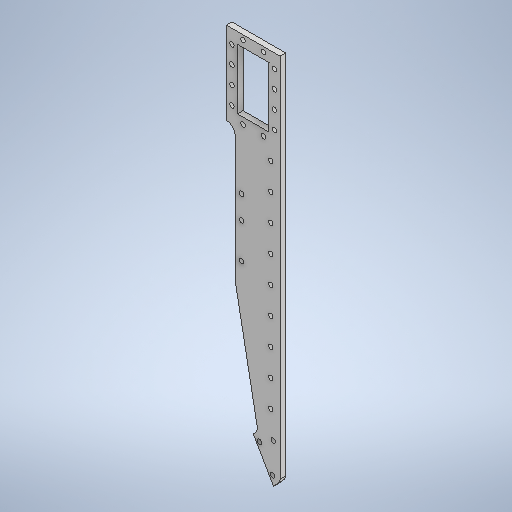
# Autodesk Inventor part: 1012
Saved by Autodesk Inventor 2025.1 (Build 291241000, 241)
## iProperties
Created: 2024-06-10
Part Number: 1012
Material: Generisch
Document SubType Name: Modeling
Designer: ffogue
Density: 1 g/cm^3
Appearance: Vorgabe
Author: ffogue
Autodesk Inventor part; units mm, degrees
ref_plane "XZ Plane" through (0, 0, 0) normal (0, 1, 0) x (-1, 0, 0)
sketch "Skizze1" plane through (0, 0, 0) normal (0, 1, 0) x (-1, 0, 0)
  line L0 (0, 0) -> (58, 0)
  line L1 (58, 0) -> (58, -89)
  arc A0 (58, -89) -> (48.5, -98.5) centre (58, -98.5) ccw
  line L2 (48.5, -98.5) -> (48.5, -218.5)
  line L3 (48.5, -218.5) -> (48.5, -234.2814)
  line L4 (0, 0) -> (0, -395.7321)
  line L5 (48.5, -218.5) -> (48.5, -250.0629) construction
  arc A1 (0, -395.7321) -> (1.4803, -399.6783) centre (6, -395.7321) ccw
  line L6 (1.4803, -399.6783) -> (7, -406)
  line L7 (7, -406) -> (29, -367.8949)
  line L8 (29, -367.8949) -> (29, -367.8949)
  arc A2 (24.7603, -358.6329) -> (29, -367.8949) centre (33.3956, -360.2814) ccw
  line L9 (24.7603, -358.6329) -> (48.5, -234.2814)
  line L10 (7, -406) -> (55.5885, -321.8422) construction
  dimension "d1" = 58
  dimension "d2" = 9.5
  dimension "d3" = 89
  dimension "d4" = 120
  dimension "d7" = 406
  dimension "d8" = 44
  dimension "d9" = 30
  dimension "d10" = 6
  dimension "d11" = 126
  dimension "d12" = 29
  dimension "d13" = 6
  constraints: 22 end point, 6 point on circle, 5 tangent, 3 centre point, 2 point on line, 2 vertical, 1 collinear, 1 horizontal, 1 midpoint, 1 parallel, 1 perpendicular
  measures "d1" distance of L0.start L0.end
  measures "d2" radius of A0
  measures "d3" distance of L0.end L1.end
  measures "d4" distance of L2.start L2.end
  measures "d7" vertical distance of L0.start L6.end
  measures "d8" distance of L6.end L7.end
  measures "d9" angle of L10 L5
  measures "d10" distance from line of A1.centre L10
  measures "d11" vertical distance of L3.end A2.centre
  measures "d12" distance from line of L4 L7.end
  measures "d13" distance from line of L4 A1.centre
extrude "Extrusion1" add sketch "Skizze1" along normal blind 6
sketch "Skizze2" plane through (0, 6, 0) normal (0, 1, 0) x (1, 0, 0)
  line L0 (-46, 12) -> (-12, 12)
  line L1 (-12, 12) -> (-12, 77)
  line L2 (-12, 77) -> (-46, 77)
  line L3 (-46, 77) -> (-46, 12)
  line L4 (-58, 0) -> (0, 0) projected
  point P0 (-29, 12)
  point P1 (-29, 0)
  dimension "d16" = 34
  dimension "d17" = 65
  dimension "d18" = 12
  constraints: 8 end point, 2 midpoint, 2 parallel, 1 horizontal, 1 perpendicular, 1 vertical alignment
  measures "d16" distance between parallel lines of L1 L3
  measures "d17" distance of L2.end L0.start
  measures "d18" distance between parallel lines of L4 L0
extrude "Extrusion2" cut sketch "Skizze2" against normal up to surface (6 mm away)
sketch "Skizze3" plane through (0, 6, 0) normal (0, 1, 0) x (1, 0, 0)
  line L0 (-58, 0) -> (0, 0) projected
  point P0 (-40, 5)
  point P1 (-18, 5)
  point P2 (-29, 0)
  point P3 (-29, 0)
  dimension "d21" = 11
  dimension "d22" = 11
  dimension "d23" = 5
  constraints: 2 midpoint, 1 horizontal alignment
  measures "d21" horizontal distance of point (-29, 0) point (-40, 5)
  measures "d22" horizontal distance of point (-29, 0) point (-18, 5)
  measures "d23" distance from line of L0 point (-18, 5)
hole "Bohrung1" at (-40, 6, -5) at (-18, 6, -5) direction (0, -1, 0) diameter 5 end through all
sketch "Skizze4" plane through (0, 6, 0) normal (0, 1, 0) x (1, 0, 0)
  circle A0 centre (-40, 5) radius 2.5 projected
  line L0 (-58, 89) -> (-58, 0) projected
  point P0 (0, 0)
  point P1 (-52, 15)
  point P2 (-52, 34)
  point P3 (-52, 53)
  point P4 (-52, 72)
  dimension "d31" = 10
  dimension "d32" = 19
  dimension "d33" = 19
  dimension "d34" = 19
  dimension "d35" = 6
  constraints: 3 vertical alignment
  measures "d31" vertical distance of point (-52, 15) A0.centre
  measures "d32" distance of point (-52, 34) point (-52, 15)
  measures "d33" distance of point (-52, 53) point (-52, 34)
  measures "d34" distance of point (-52, 72) point (-52, 53)
  measures "d35" distance from line of point (-52, 15) L0
hole "Bohrung2" at (-52, 6, -15) at (-52, 6, -34) at (-52, 6, -53) at (-52, 6, -72) direction (0, -1, 0) diameter 5 depth 6
ref_plane "Arbeitsebene1" through (-29, 0, 0) normal (1, 0, 0) x (0, 1, 0)
mirror "Spiegeln1" about plane through (-29, 0, 0) normal (1, 0, 0) of "Bohrung2"
ref_plane "Arbeitsebene2" through (0, 0, -44.5) normal (0, 0, 1) x (1, 0, 0)
mirror "Spiegeln2" about plane through (0, 0, -44.5) normal (0, 0, 1) of "Bohrung1"
sketch "Skizze5" plane through (0, 6, 0) normal (0, 1, 0) x (1, 0, 0)
  circle A0 centre (-18, 84) radius 2.5 projected
  line L0 (0, 0) -> (0, 395.7321) projected
  point P0 (-10, 103)
  point P1 (-10, 132)
  point P2 (-10, 161)
  point P3 (-10, 190)
  point P4 (-10, 277)
  point P5 (-10, 306)
  point P6 (-10, 335)
  point P7 (-10, 219)
  point P8 (-10, 248)
  dimension "d45" = 19
  dimension "d46" = 29
  dimension "d47" = 29
  dimension "d48" = 29
  dimension "d49" = 29
  dimension "d50" = 29
  dimension "d51" = 29
  dimension "d52" = 29
  dimension "d53" = 29
  dimension "d54" = 10
  constraints: 8 vertical alignment
  measures "d45" vertical distance of point (-10, 103) A0.centre
  measures "d46" distance of point (-10, 132) point (-10, 103)
  measures "d47" distance of point (-10, 161) point (-10, 132)
  measures "d48" distance of point (-10, 190) point (-10, 161)
  measures "d49" distance of point (-10, 219) point (-10, 190)
  measures "d50" distance of point (-10, 335) point (-10, 306)
  measures "d51" distance of point (-10, 306) point (-10, 277)
  measures "d52" distance of point (-10, 277) point (-10, 248)
  measures "d53" distance of point (-10, 248) point (-10, 219)
  measures "d54" distance from line of L0 point (-10, 335)
hole "Bohrung3" at (-10, 6, -103) at (-10, 6, -132) at (-10, 6, -161) at (-10, 6, -190) at (-10, 6, -277) at (-10, 6, -306) at (-10, 6, -335) at (-10, 6, -219) at (-10, 6, -248) direction (0, -1, 0) diameter 5 depth 6
sketch "Skizze6" plane through (0, 6, 0) normal (0, 1, 0) x (1, 0, 0)
  arc A0 (-58, 89) -> (-48.5, 98.5) centre (-58, 98.5) ccw projected
  line L0 (-48.5, 234.2814) -> (-48.5, 98.5) projected
  point P0 (0, 0)
  point P1 (-41.5, 149.5)
  point P2 (-41.5, 174.5)
  point P3 (-41.5, 212.5)
  dimension "d62" = 51
  dimension "d63" = 25
  dimension "d64" = 38
  dimension "d65" = 7
  constraints: 2 vertical alignment
  measures "d62" vertical distance of point (-41.5, 149.5) A0.centre
  measures "d63" distance of point (-41.5, 174.5) point (-41.5, 149.5)
  measures "d64" distance of point (-41.5, 212.5) point (-41.5, 174.5)
  measures "d65" distance from line of L0 point (-41.5, 149.5)
hole "Bohrung4" at (-41.5, 6, -149.5) at (-41.5, 6, -174.5) at (-41.5, 6, -212.5) direction (0, -1, 0) diameter 5 depth 6
sketch "Skizze8" plane through (0, 6, 0) normal (0, 1, 0) x (1, 0, 0)
  line L0 (-7, 406) -> (-29, 367.8949) projected
  line L1 (-4.2402, 402.8391) -> (-26.0353, 365.0889) construction
  arc A0 (-24.7603, 358.6329) -> (-29, 367.8949) centre (-33.3956, 360.2814) ccw projected
  line L2 (-1.4803, 399.6783) -> (-7, 406) projected
  line L3 (-15.1377, 383.964) -> (-49.9282, 404.0503) construction
  line L4 (-22.1377, 371.8397) -> (-7.4153, 363.3397) construction
  point P0 (0, 0)
  point P1 (-8.1377, 396.0884)
  dimension "d90" = 90
  dimension "d91" = 14
  dimension "d92" = 28
  dimension "d93" = 90
  dimension "d94" = 17
  constraints: 6 end point, 2 midpoint, 2 point on line, 1 parallel, 1 point on circle
  measures "d90" angle of L1 L3
  measures "d91" distance from line of L3 L4.start
  measures "d92" distance of point (-8.138, 396.088) L4.start
  measures "d93" angle of L4 L1
  measures "d94" distance of L4.start L4.end
hole "Bohrung5" at (-7.4153, 6, -363.3397) at (-22.1377, 6, -371.8397) at (-8.1377, 6, -396.0884) direction (0, -1, 0) diameter 4.917 depth 6 thread size "M6x1" class "6H" standard "ISO Metric profile"
equation "\"d22\" = d21"
equation "\"d33\" = d32"
equation "\"d34\" = d33"
equation "\"d47\" = d46"
equation "\"d48\" = d46"
equation "\"d49\" = d46"
equation "\"d50\" = d46"
equation "\"d51\" = d46"
equation "\"d52\" = d46"
equation "\"d53\" = d46"
